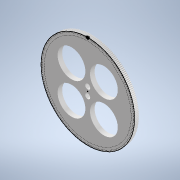
# Autodesk Inventor part: horizontal_axis_big_gear
Saved by Autodesk Inventor 2021 (Build 250183000, 183)
## iProperties
Created: 2020-10-04
Part Number: horizontal_axis_big_gear
Material: Generic
Document SubType Name: Modeling
Designer: bober
Density: 1 g/cm^3
Appearance: Default
Author: bober
Autodesk Inventor part; units mm, degrees
ref_plane "YZ Plane" through (0, 0, 0) normal (1, 0, 0) x (0, 1, 0)
ref_plane "XZ Plane" through (0, 0, 0) normal (0, 1, 0) x (-1, 0, 0)
ref_plane "XY Plane" through (0, 0, 0) normal (0, 0, 1) x (1, 0, 0)
sketch "Sketch1" plane through (0, 0, 0) normal (0, 0, 1) x (1, 0, 0)
  spline S0 degree 3 poles (-1.2656, 100.9921) (-1.1744, 100.7653) (-0.9921, 100.3117) (-0.7787, 99.7392) (-0.6166, 99.278) (-0.5147, 98.9901) (-0.458, 98.7994) (-0.4209, 98.7155) (-0.3986, 98.6754) (-0.3711, 98.6386) (-0.3402, 98.6046) (-0.3051, 98.575) (-0.267, 98.5494) (-0.2257, 98.5291) (-0.1823, 98.5143) (-0.1375, 98.5042) (-0.0764, 98.5001) (0, 98.5024) (0.0764, 98.5001) (0.1375, 98.5042) (0.1823, 98.5143) (0.2257, 98.5291) (0.267, 98.5494) (0.3051, 98.575) (0.3402, 98.6046) (0.3711, 98.6386) (0.3986, 98.6754) (0.4209, 98.7155) (0.458, 98.7994) (0.5147, 98.9901) (0.6166, 99.278) (0.7787, 99.7392) (0.9921, 100.3117) (1.1744, 100.7653) (1.2656, 100.9921) knots 0 0 0 0 0.07332 0.14664 0.1833 0.219961 0.238288 0.242867 0.247449 0.252032 0.256612 0.261194 0.265775 0.270356 0.274938 0.279519 0.284099 0.293264 0.30243 0.307009 0.311591 0.316173 0.320754 0.325335 0.329917 0.334497 0.33908 0.343662 0.348241 0.366568 0.403229 0.439889 0.513209 0.586529 0.586529 0.586529 0.586529
  circle A0 centre (0, 0) radius 98.5015 construction
  circle A1 centre (0, 0) radius 93.9693 construction
  circle A2 centre (0, 0) radius 100 construction
  circle A3 centre (0, 0) radius 101
  point P0 (-0.995, 100.3106)
  point P1 (-0.7389, 99.6236)
  point P2 (-0.6165, 99.2781)
  point P3 (-0.4982, 98.931)
  point P4 (-0.4391, 98.7576)
  point P5 (-0.4203, 98.7158)
  point P6 (-0.3977, 98.6759)
  point P7 (-0.3705, 98.6391)
  point P8 (-0.3395, 98.6053)
  point P9 (-0.3046, 98.5756)
  point P10 (-0.2665, 98.5503)
  point P11 (-0.2254, 98.53)
  point P12 (-0.1821, 98.5151)
  point P13 (-0.1373, 98.5053)
  point P14 (-0.0917, 98.5016)
  point P15 (0, 98.5015)
  point P16 (0.0917, 98.5016)
  point P17 (0.1373, 98.5053)
  point P18 (0.1821, 98.5151)
  point P19 (0.2254, 98.53)
  point P20 (0.2665, 98.5503)
  point P21 (0.3046, 98.5756)
  point P22 (0.3395, 98.6053)
  point P23 (0.3705, 98.6391)
  point P24 (0.3977, 98.6759)
  point P25 (0.4203, 98.7158)
  point P26 (0.4391, 98.7576)
  point P27 (0.4982, 98.931)
  point P28 (0.6165, 99.2781)
  point P29 (0.7389, 99.6236)
  point P30 (0.995, 100.3106)
  constraints: 4 centre point, 2 point on circle, 71 other
extrude "Extrusion1" add sketch "Sketch1" against normal blind 10
extrude "Extrusion2" cut sketch "Sketch1" against normal blind 10 contours A3 S0 picked at (-0.0238, 99.8482)
pattern_circular "Circular Pattern1" count 200 over 360 about axis through (0, 0, 0) along (0, 0, -1) of "Extrusion2"
sketch "Sketch2" plane through (0, 0, 0) normal (0, 0, 1) x (1, 0, 0)
  circle A0 centre (0, 9) radius 5.45
  circle A1 centre (0, -9) radius 5.45
  point P0 (0, 0)
  dimension "d7" = 10.9
  dimension "d8" = 10.9
  constraints: 2 centre point
  measures "d7" diameter of A0
  measures "d8" diameter of A1
extrude "Extrusion3" cut sketch "Sketch2" against normal blind 10
sketch "Sketch3" plane through (0, 0, 0) normal (0, 0, 1) x (1, 0, 0)
  line L0 (-35, 35) -> (35, 35)
  line L1 (35, 35) -> (35, -35)
  line L2 (35, -35) -> (-35, -35)
  line L3 (-35, -35) -> (-35, 35)
  line L4 (-35, 35) -> (35, -35) construction
  line L5 (35, 35) -> (-35, -35) construction
  point P0 (0, 0)
  dimension "d11" = 70
  dimension "d12" = 70
  constraints: 12 end point, 2 midpoint, 2 parallel, 1 horizontal, 1 perpendicular
  measures "d11" distance of L1.end L2.end
  measures "d12" distance of L0.end L1.end
hole "Hole1" at (-35, 35, 0) at (35, 35, 0) at (35, -35, 0) at (-35, -35, 0) direction (0, 0, -1) diameter 60 end through all
sketch "Sketch4" plane through (0, 0, 0) normal (0, 0, 1) x (1, 0, 0)
  point P0 (0, 0)
sketch "Sketch5" plane through (0, 0, -10) normal (0, 0, -1) x (-1, 0, 0)
  point P0 (0, 0)
  point P1 (0, 0)
  constraints: 1 coincident
equation "\"d0\" = FaceWidth"
equation "\"Module\" = 1"
equation "\"PressureAngle\" = 20deg"
equation "\"UnitProfileClearance\" = 0.25"
equation "\"UnitRoundRadius\" = 0.35"
equation "\"HeadDiameter\" = 202"
equation "\"RootDiameter\" = 197.00295"
equation "\"BaseDiameter\" = 187.93852"
equation "\"FaceWidth\" = 10"
equation "\"HelixAngle\" = 0"
equation "\"UnitCorrection\" = 0"
equation "\"UnitAddendumModification\" = 0"
equation "\"CircularPitch\" = 3.141593"
equation "\"UnitBacklashShift\" = -0.248523"
equation "\"TotalToolShift\" = -0.24852"
equation "\"IsInternal\" = 0"
body "Solid1"
